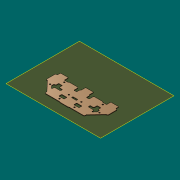
# Autodesk Inventor part: Part2
Saved by Autodesk Inventor 2018 (Build 220112000, 112)
## iProperties
Created: 2021-10-17
Part Number: Part2
Material: アルミニウム 6061
Document SubType Name: Modeling
Designer: gisen
Density: 2.7 g/cm^3
Appearance: アルミニウム - フラット
Author: gisen
Autodesk Inventor part; units mm, degrees
ref_plane "YZ Plane" through (0, 0, 0) normal (1, 0, 0) x (0, 1, 0)
ref_plane "XZ Plane" through (0, 0, 0) normal (0, 1, 0) x (-1, 0, 0)
ref_plane "XY Plane" through (0, 0, 0) normal (0, 0, 1) x (1, 0, 0)
ref_plane "作業平面1" through (0, -39.175, 8.3) normal (0, 0, -1) x (-1, 0, 0)
sketch "スケッチ1" plane through (0, -39.175, 8.3) normal (0, 0, -1) x (-1, 0, 0)
  arc A0 (-5.35, 6.375) -> (-6.35, 5.375) centre (-5.35, 5.375) ccw construction
  arc A1 (6.35, 5.375) -> (5.35, 6.375) centre (5.35, 5.375) ccw construction
  arc A2 (-32.9, 5.375) -> (-33.9, 6.375) centre (-33.9, 5.375) ccw construction
  arc A3 (-44.6, 6.375) -> (-45.6, 5.375) centre (-44.6, 5.375) ccw construction
  arc A4 (33.9, 6.375) -> (32.9, 5.375) centre (33.9, 5.375) ccw construction
  arc A5 (45.6, 5.375) -> (44.6, 6.375) centre (44.6, 5.375) ccw construction
  arc A6 (48.3, -0.325) -> (46.5, 1.475) centre (46.5, -0.325) ccw construction
  arc A7 (46.5, -13.925) -> (48.3, -12.125) centre (46.5, -12.125) ccw construction
  arc A8 (-46.5, 1.475) -> (-48.3, -0.325) centre (-46.5, -0.325) ccw construction
  arc A9 (-48.3, -12.125) -> (-46.5, -13.925) centre (-46.5, -12.125) ccw construction
  arc A10 (-17.5, -33.025) -> (-15.7, -31.225) centre (-17.5, -31.225) ccw construction
  arc A11 (15.7, -31.225) -> (17.5, -33.025) centre (17.5, -31.225) ccw construction
  arc A12 (31.1, -19.425) -> (29.3, -17.625) centre (29.3, -19.425) ccw construction
  arc A13 (-5.9, -0.585) -> (-7.7, -2.385) centre (-5.9, -2.385) ccw construction
  arc A14 (7.7, -2.385) -> (5.9, -0.585) centre (5.9, -2.385) ccw construction
  arc A15 (13.6, 0.875) -> (12.2994, 0.3193) centre (13.6, -0.925) ccw construction
  arc A16 (27.2, -0.925) -> (25.4, 0.875) centre (25.4, -0.925) ccw construction
  arc A17 (34.7, 1.475) -> (32.9, -0.325) centre (34.7, -0.325) ccw construction
  arc A18 (-12.2994, 0.3193) -> (-13.6, 0.875) centre (-13.6, -0.925) ccw construction
  arc A19 (-25.4, 0.875) -> (-27.2, -0.925) centre (-25.4, -0.925) ccw construction
  arc A20 (-32.9, -0.325) -> (-34.7, 1.475) centre (-34.7, -0.325) ccw construction
  arc A21 (-13.6, -14.525) -> (-11.8, -12.725) centre (-13.6, -12.725) ccw construction
  arc A22 (-3.25, -15.985) -> (-3.75, -16.485) centre (-3.25, -16.485) ccw construction
  arc A23 (-3.75, -17.725) -> (-3.25, -18.225) centre (-3.25, -17.725) ccw construction
  arc A24 (3.75, -16.485) -> (3.25, -15.985) centre (3.25, -16.485) ccw construction
  arc A25 (3.25, -18.225) -> (3.75, -17.725) centre (3.25, -17.725) ccw construction
  arc A26 (-15.7, -25.525) -> (-15.2, -26.025) centre (-15.2, -25.525) ccw construction
  arc A27 (-8.2, -26.025) -> (-7.7, -25.525) centre (-8.2, -25.525) ccw construction
  arc A28 (-15.2, -21.625) -> (-15.7, -22.125) centre (-15.2, -22.125) ccw construction
  arc A29 (-7.7, -22.125) -> (-8.2, -21.625) centre (-8.2, -22.125) ccw construction
  arc A30 (-7.317, -32.935) -> (-5.9, -33.625) centre (-5.9, -31.825) ccw construction
  arc A31 (5.9, -33.625) -> (7.317, -32.935) centre (5.9, -31.825) ccw construction
  line L0 (-7.4492, -33.025) -> (-17.5, -33.025) construction
  line L1 (17.5, -33.025) -> (7.4492, -33.025) construction
  line L2 (-31.306, -29.2915) -> (-45.7404, -14.0808) construction
  line L3 (45.7404, -14.0808) -> (31.306, -29.2915) construction
  arc A32 (-46.1, 1.475) -> (-45.6, 1.975) centre (-46.1, 1.975) ccw construction
  line L4 (-46.5, 1.375) -> (-46.1, 1.375)
  line L5 (-45.5, 1.975) -> (-45.5, 5.375)
  line L6 (-44.6, 6.275) -> (-33.9, 6.275)
  line L7 (-33, 5.375) -> (-33, 0.275)
  line L8 (-32.4, -0.325) -> (-27.3621, -0.325)
  arc A33 (-27.3621, -0.325) -> (-26.8503, -0.038) centre (-27.3621, 0.275) ccw
  arc A34 (-25.4, 0.775) -> (-26.8503, -0.038) centre (-25.4, -0.925) ccw
  line L9 (-25.4, 0.775) -> (-13.6, 0.775)
  line L10 (-11.9, -0.925) -> (-11.9, -5.875)
  line L11 (-11.3, -6.475) -> (-8.2, -6.475)
  line L12 (-7.6, -5.875) -> (-7.6, -2.385)
  arc A35 (-6.8321, -0.8452) -> (-6.35, 0.0103) centre (-7.35, 0.0103) ccw construction
  arc A36 (-6.7804, -0.9307) -> (-7.6, -2.385) centre (-5.9, -2.385) ccw
  arc A37 (-6.7804, -0.9307) -> (-6.25, 0.0103) centre (-7.35, 0.0103) ccw
  line L13 (-6.25, 0.0103) -> (-6.25, 5.375)
  line L14 (-5.35, 6.275) -> (5.35, 6.275)
  arc A38 (-5.35, 6.275) -> (-6.25, 5.375) centre (-5.35, 5.375) ccw
  arc A39 (-33, 5.375) -> (-33.9, 6.275) centre (-33.9, 5.375) ccw
  arc A40 (-44.6, 6.275) -> (-45.5, 5.375) centre (-44.6, 5.375) ccw
  arc A41 (-46.1, 1.375) -> (-45.5, 1.975) centre (-46.1, 1.975) ccw
  arc A42 (-33, 0.275) -> (-32.4, -0.325) centre (-32.4, 0.275) ccw
  arc A43 (-11.9, -5.875) -> (-11.3, -6.475) centre (-11.3, -5.875) ccw
  arc A44 (-8.2, -6.475) -> (-7.6, -5.875) centre (-8.2, -5.875) ccw
  arc A45 (-11.8, -5.875) -> (-11.3, -6.375) centre (-11.3, -5.875) ccw construction
  arc A46 (-8.2, -6.375) -> (-7.7, -5.875) centre (-8.2, -5.875) ccw construction
  arc A47 (-11.9, -0.925) -> (-13.6, 0.775) centre (-13.6, -0.925) ccw
  arc A48 (-32.9, 0.275) -> (-32.4, -0.225) centre (-32.4, 0.275) ccw construction
  arc A49 (-27.3621, -0.225) -> (-26.9356, 0.0141) centre (-27.3621, 0.275) ccw construction
  line L15 (-48.2, -0.325) -> (-48.2, -12.125)
  arc A50 (-48.2, -12.125) -> (-46.5, -13.825) centre (-46.5, -12.125) ccw
  line L16 (-45.6678, -14.012) -> (-31, -29.4687)
  arc A51 (-46.5, 1.375) -> (-48.2, -0.325) centre (-46.5, -0.325) ccw
  arc A52 (-45.7404, -14.0808) -> (-46.1031, -13.925) centre (-46.1031, -14.425) ccw construction
  line L17 (-17.5, -33.025) -> (-29.25, -33.025) construction
  line L18 (-31, -29.4687) -> (-31, -31.6478)
  line L19 (-31, -31.6478) -> (-29.788, -32.925)
  line L20 (-32.394, -30.324) -> (-30.1373, -32.7021) construction
  line L21 (-3.25, -15.985) -> (3.25, -15.985) construction
  line L22 (3.25, -18.225) -> (-3.25, -18.225) construction
  line L23 (0, -15.985) -> (0, -18.225) construction
  arc A53 (-35.492, -17.4172) -> (-35.3547, -17.7614) centre (-34.992, -17.4172) ccw construction
  line L24 (-32.1208, -21.1692) -> (-35.3547, -17.7614) construction
  arc A54 (-32.1208, -21.1692) -> (-31.7581, -21.325) centre (-31.7581, -20.825) ccw construction
  line L25 (-31.6, -21.325) -> (-31.7581, -21.325) construction
  arc A55 (-31.6, -21.325) -> (-31.1, -20.825) centre (-31.6, -20.825) ccw construction
  line L26 (-31.1, -19.425) -> (-31.1, -20.825) construction
  arc A56 (-29.3, -17.625) -> (-31.1, -19.425) centre (-29.3, -19.425) ccw construction
  line L27 (-22.2, -17.625) -> (-29.3, -17.625) construction
  arc A57 (-22.2, -17.625) -> (-21.7, -17.125) centre (-22.2, -17.125) ccw construction
  line L28 (-21.7, -15.025) -> (-21.7, -17.125) construction
  arc A58 (-21.7, -15.025) -> (-22.2, -14.525) centre (-22.2, -15.025) ccw construction
  line L29 (-25.4, -14.525) -> (-22.2, -14.525) construction
  arc A59 (-27.2, -12.725) -> (-25.4, -14.525) centre (-25.4, -12.725) ccw construction
  line L30 (-27.2, -9.725) -> (-27.2, -12.725) construction
  arc A60 (-27.2, -9.725) -> (-27.7, -9.225) centre (-27.7, -9.725) ccw construction
  line L31 (-32.4, -9.225) -> (-27.7, -9.225) construction
  arc A61 (-32.4, -9.225) -> (-32.9, -9.725) centre (-32.4, -9.725) ccw construction
  line L32 (-32.9, -12.125) -> (-32.9, -9.725) construction
  arc A62 (-34.7, -13.925) -> (-32.9, -12.125) centre (-34.7, -12.125) ccw construction
  line L33 (-34.992, -13.925) -> (-34.7, -13.925) construction
  arc A63 (-34.992, -13.925) -> (-35.492, -14.425) centre (-34.992, -14.425) ccw construction
  line L34 (-35.492, -17.4172) -> (-35.492, -14.425) construction
  arc A64 (-27.1, -9.725) -> (-27.7, -9.125) centre (-27.7, -9.725) ccw
  line L35 (-27.1, -9.725) -> (-27.1, -12.725)
  arc A65 (-27.1, -12.725) -> (-25.4, -14.425) centre (-25.4, -12.725) ccw
  line L36 (-25.4, -14.425) -> (-22.2, -14.425)
  arc A66 (-21.6, -15.025) -> (-22.2, -14.425) centre (-22.2, -15.025) ccw
  line L37 (-21.6, -15.025) -> (-21.6, -17.125)
  arc A67 (-22.2, -17.725) -> (-21.6, -17.125) centre (-22.2, -17.125) ccw
  line L38 (-22.2, -17.725) -> (-29.3, -17.725)
  arc A68 (-29.3, -17.725) -> (-31, -19.425) centre (-29.3, -19.425) ccw
  line L39 (-31, -19.425) -> (-31, -20.825)
  arc A69 (-31.6, -21.425) -> (-31, -20.825) centre (-31.6, -20.825) ccw
  line L40 (-31.6, -21.425) -> (-31.7581, -21.425)
  arc A70 (-32.1933, -21.238) -> (-31.7581, -21.425) centre (-31.7581, -20.825) ccw
  line L41 (-32.1933, -21.238) -> (-35.4272, -17.8302)
  arc A71 (-35.592, -17.4172) -> (-35.4272, -17.8302) centre (-34.992, -17.4172) ccw
  line L42 (-35.592, -17.4172) -> (-35.592, -14.425)
  arc A72 (-34.992, -13.825) -> (-35.592, -14.425) centre (-34.992, -14.425) ccw
  line L43 (-34.992, -13.825) -> (-34.7, -13.825)
  arc A73 (-34.7, -13.825) -> (-33, -12.125) centre (-34.7, -12.125) ccw
  line L44 (-33, -12.125) -> (-33, -9.725)
  arc A74 (-32.4, -9.125) -> (-33, -9.725) centre (-32.4, -9.725) ccw
  line L45 (-32.4, -9.125) -> (-27.7, -9.125)
  line L46 (-15.2, -21.525) -> (-8.2, -21.525)
  line L47 (-7.6, -22.125) -> (-7.6, -25.525)
  line L48 (-8.2, -26.125) -> (-15.2, -26.125)
  line L49 (-15.8, -25.525) -> (-15.8, -22.125)
  line L50 (-3.25, -15.885) -> (3.25, -15.885)
  line L51 (3.85, -16.485) -> (3.85, -17.725)
  line L52 (3.25, -18.325) -> (-3.25, -18.325)
  line L53 (-3.85, -17.725) -> (-3.85, -16.485)
  arc A75 (-15.2, -21.525) -> (-15.8, -22.125) centre (-15.2, -22.125) ccw
  arc A76 (-7.6, -22.125) -> (-8.2, -21.525) centre (-8.2, -22.125) ccw
  arc A77 (-8.2, -26.125) -> (-7.6, -25.525) centre (-8.2, -25.525) ccw
  arc A78 (-15.8, -25.525) -> (-15.2, -26.125) centre (-15.2, -25.525) ccw
  arc A79 (-3.85, -17.725) -> (-3.25, -18.325) centre (-3.25, -17.725) ccw
  arc A80 (-3.25, -15.885) -> (-3.85, -16.485) centre (-3.25, -16.485) ccw
  arc A81 (3.85, -16.485) -> (3.25, -15.885) centre (3.25, -16.485) ccw
  arc A82 (3.25, -18.325) -> (3.85, -17.725) centre (3.25, -17.725) ccw
  line L54 (-29.788, -32.925) -> (-7.1961, -32.925)
  arc A83 (-7.1961, -32.925) -> (-5.9, -33.525) centre (-5.9, -31.825) ccw
  line L55 (-5.9, -33.525) -> (5.9, -33.525)
  line L56 (-5.9, -33.625) -> (5.9, -33.625) construction
  line L57 (-46.5, -13.825) -> (-46.1031, -13.825)
  arc A84 (-45.6678, -14.012) -> (-46.1031, -13.825) centre (-46.1031, -14.425) ccw
  line L58 (46.5, 1.375) -> (46.1, 1.375)
  line L59 (45.5, 1.975) -> (45.5, 5.375)
  line L60 (44.6, 6.275) -> (33.9, 6.275)
  line L61 (33, 5.375) -> (33, 0.275)
  line L62 (32.4, -0.325) -> (27.3621, -0.325)
  arc A85 (26.8503, -0.038) -> (27.3621, -0.325) centre (27.3621, 0.275) ccw
  arc A86 (26.8503, -0.038) -> (25.4, 0.775) centre (25.4, -0.925) ccw
  line L63 (25.4, 0.775) -> (13.6, 0.775)
  line L64 (11.9, -0.925) -> (11.9, -5.875)
  line L65 (11.3, -6.475) -> (8.2, -6.475)
  line L66 (7.6, -5.875) -> (7.6, -2.385)
  arc A87 (7.6, -2.385) -> (6.7804, -0.9307) centre (5.9, -2.385) ccw
  arc A88 (6.25, 0.0103) -> (6.7804, -0.9307) centre (7.35, 0.0103) ccw
  line L67 (6.25, 0.0103) -> (6.25, 5.375)
  arc A89 (6.25, 5.375) -> (5.35, 6.275) centre (5.35, 5.375) ccw
  arc A90 (33.9, 6.275) -> (33, 5.375) centre (33.9, 5.375) ccw
  arc A91 (45.5, 5.375) -> (44.6, 6.275) centre (44.6, 5.375) ccw
  arc A92 (45.5, 1.975) -> (46.1, 1.375) centre (46.1, 1.975) ccw
  arc A93 (32.4, -0.325) -> (33, 0.275) centre (32.4, 0.275) ccw
  arc A94 (11.3, -6.475) -> (11.9, -5.875) centre (11.3, -5.875) ccw
  arc A95 (7.6, -5.875) -> (8.2, -6.475) centre (8.2, -5.875) ccw
  arc A96 (13.6, 0.775) -> (11.9, -0.925) centre (13.6, -0.925) ccw
  line L68 (48.2, -0.325) -> (48.2, -12.125)
  arc A97 (46.5, -13.825) -> (48.2, -12.125) centre (46.5, -12.125) ccw
  line L69 (45.6678, -14.012) -> (31, -29.4687)
  arc A98 (48.2, -0.325) -> (46.5, 1.375) centre (46.5, -0.325) ccw
  line L70 (31, -29.4687) -> (31, -31.6478)
  line L71 (31, -31.6478) -> (29.788, -32.925)
  arc A99 (27.7, -9.125) -> (27.1, -9.725) centre (27.7, -9.725) ccw
  line L72 (27.1, -9.725) -> (27.1, -12.725)
  arc A100 (25.4, -14.425) -> (27.1, -12.725) centre (25.4, -12.725) ccw
  line L73 (25.4, -14.425) -> (22.2, -14.425)
  arc A101 (22.2, -14.425) -> (21.6, -15.025) centre (22.2, -15.025) ccw
  line L74 (21.6, -15.025) -> (21.6, -17.125)
  arc A102 (21.6, -17.125) -> (22.2, -17.725) centre (22.2, -17.125) ccw
  line L75 (22.2, -17.725) -> (29.3, -17.725)
  arc A103 (31, -19.425) -> (29.3, -17.725) centre (29.3, -19.425) ccw
  line L76 (31, -19.425) -> (31, -20.825)
  arc A104 (31, -20.825) -> (31.6, -21.425) centre (31.6, -20.825) ccw
  line L77 (31.6, -21.425) -> (31.7581, -21.425)
  arc A105 (31.7581, -21.425) -> (32.1933, -21.238) centre (31.7581, -20.825) ccw
  line L78 (32.1933, -21.238) -> (35.4272, -17.8302)
  arc A106 (35.4272, -17.8302) -> (35.592, -17.4172) centre (34.992, -17.4172) ccw
  line L79 (35.592, -17.4172) -> (35.592, -14.425)
  arc A107 (35.592, -14.425) -> (34.992, -13.825) centre (34.992, -14.425) ccw
  line L80 (34.992, -13.825) -> (34.7, -13.825)
  arc A108 (33, -12.125) -> (34.7, -13.825) centre (34.7, -12.125) ccw
  line L81 (33, -12.125) -> (33, -9.725)
  arc A109 (33, -9.725) -> (32.4, -9.125) centre (32.4, -9.725) ccw
  line L82 (32.4, -9.125) -> (27.7, -9.125)
  line L83 (15.2, -21.525) -> (8.2, -21.525)
  line L84 (7.6, -22.125) -> (7.6, -25.525)
  line L85 (8.2, -26.125) -> (15.2, -26.125)
  line L86 (15.8, -25.525) -> (15.8, -22.125)
  arc A110 (15.8, -22.125) -> (15.2, -21.525) centre (15.2, -22.125) ccw
  arc A111 (8.2, -21.525) -> (7.6, -22.125) centre (8.2, -22.125) ccw
  arc A112 (7.6, -25.525) -> (8.2, -26.125) centre (8.2, -25.525) ccw
  arc A113 (15.2, -26.125) -> (15.8, -25.525) centre (15.2, -25.525) ccw
  line L87 (29.788, -32.925) -> (7.1961, -32.925)
  arc A114 (5.9, -33.525) -> (7.1961, -32.925) centre (5.9, -31.825) ccw
  line L88 (46.5, -13.825) -> (46.1031, -13.825)
  arc A115 (46.1031, -13.825) -> (45.6678, -14.012) centre (46.1031, -14.425) ccw
  circle A116 centre (-38.492, -16.925) radius 0.8 construction
  circle A117 centre (-11.7, -29.025) radius 0.8 construction
  circle A118 centre (-9.75, -16.375) radius 0.8 construction
  circle A119 centre (-30.05, -3.225) radius 0.8 construction
  circle A120 centre (9.75, -16.375) radius 0.8 construction
  circle A121 centre (11.7, -29.025) radius 0.8 construction
  circle A122 centre (38.492, -16.925) radius 0.8 construction
  circle A123 centre (30.05, -3.225) radius 0.8 construction
  circle A124 centre (-30.05, -3.225) radius 1.05
  circle A125 centre (-38.492, -16.925) radius 1.05
  circle A126 centre (-11.7, -29.025) radius 1.05
  circle A127 centre (-9.75, -16.375) radius 1.05
  circle A128 centre (9.75, -16.375) radius 1.05
  circle A129 centre (11.7, -29.025) radius 1.05
  circle A130 centre (38.492, -16.925) radius 1.05
  circle A131 centre (30.05, -3.225) radius 1.05
  point P0 (0, 39.175)
  point P1 (-31.1, -29.8078)
  dimension "d1" = 0.1
  dimension "d9" = 0.1
  dimension "d10" = 0.1
  dimension "d11" = 0.1
  dimension "d13" = 0.1
  dimension "d14" = 0.1
  dimension "d15" = 2.1
  dimension "d18" = 0.1
  constraints: 142 end point, 132 point on circle, 94 symmetric about line, 74 centre point, 45 tangent, 29 coincident, 19 equal radius, 9 perpendicular, 8 horizontal, 7 parallel, 4 vertical, 2 midpoint, 55 other
  measures "d1" distance from line of A0.start L14
  measures "d9" distance from line of L17 L19.end
  measures "d10" distance from line of L20 L18.end
  measures "d11" distance between parallel lines of L45 L31
  measures "d13" distance from line of A28.start L46
  measures "d14" distance between parallel lines of L55 L56
  measures "d15" diameter of A124
  measures "d18" distance from line of point (-31.1, -29.808) L18
extrude "押し出し1" add sketch "スケッチ1" along normal blind 0.8
equation "\"d9\" = d1"
equation "\"d10\" = d1"
equation "\"d11\" = d1"
equation "\"d13\" = d1"
equation "\"d14\" = d1"
equation "\"d18\" = d1"
